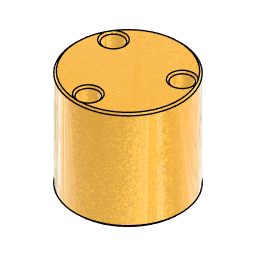
Parametric Starkiller v5 (Autodesk Fusion 360 design; units mm, degrees)
Autodesk Fusion 360 part; units mm, degrees
sketch "Sketch1" plane through (0, 0, 0) normal (0, 0, 1) x (1, 0, 0)
  circle A0 centre (0, 0) radius 11.7
  dimension "d18" = 23.4
  constraint coincident A0.centre origin
  measures "d18" diameter of A0
extrude "Main body contour" add sketch "Sketch1" along normal blind 22
sketch "bottom circle" plane through (0, 0, 0) normal (0, 0, -1) x (1, 0, 0)
  circle A0 centre (0, 0) radius 11.7
  circle A1 centre (0, 0) radius 5.69
  dimension "d21" = 11.38
  constraint concentric A0 A1
  measures "d21" diameter of A1
ref_plane "WorkPlane1" through (0, 0, 22) normal (0, 0, 1) x (1, 0, 0)
extrude "bottom hole" cut sketch "bottom circle" against normal blind 6.4 contours A1
sketch "Sketch3" plane through (0, 0, 22) normal (0, 0, 1) x (1, 0, 0)
  circle A0 centre (0, 0) radius 11.7 construction
  line L0 (0, 0) -> (0, -8.85) construction
  circle A1 centre (0, -8.85) radius 2.1
  circle A2 centre (0, 0) radius 12.6 construction
  circle A3 centre (0, 0) radius 5.1 construction
  circle A4 centre (0, -8.85) radius 3.75 construction
  dimension "d25" = 4.2
  dimension "d50" = 25.2
  dimension "d51" = 10.2
  constraint coincident A0.centre L0.start
  constraint vertical L0
  constraint coincident L0.end A1.centre
  constraint concentric A0 A3
  constraint concentric A1 A4
  constraint tangent A2 A4
  constraint tangent A3 A4
  measures "d25" diameter of A1
  measures "d50" diameter of A2
  measures "d51" diameter of A3
extrude "Extrude3" cut sketch "Sketch3" against normal blind 6.4
pattern_circular "C-Pattern1" count 3 over 360 about axis through (0, 0, 1.75) along (0, 0, 1) of "Extrude3"
sketch "Sketch4" plane through (0, 0, 0) normal (0, 0, -1) x (1, 0, 0)
  circle A0 centre (0, 0) radius 5.69
  circle A1 centre (0, 0) radius 11.7
  line L0 (0, 0) -> (0, 5.69) construction
  line L1 (-0.4202, 5.6745) -> (0, 5.29)
  line L2 (0, 5.29) -> (0.4202, 5.6745)
  line L3 (-0.4202, 5.6745) -> (0, 0) construction
  line L4 (0, 0) -> (0.4202, 5.6745) construction
  dimension "d34" = 0.4
  dimension "d43" = 8.471
  constraint coincident A0.centre A1.centre
  constraint coincident A0 L0.end
  constraint vertical L0
  constraint coincident A0 L1.start
  constraint coincident L0 L1.end
  constraint coincident A0 L2.end
  constraint equal L1 L2
  measures "d34" distance of L0.end L1.end
  measures "d43" angle of L3 L4
extrude "Extrude4" add sketch "Sketch4" against normal blind 6.4 contours A0 L1 L2 picked at (0, 5.5555)
sketch "Sketch5" plane through (0, 0, 0) normal (1, 0, 0) x (0, 1, 0)
  line L0 (-5.6745, 6.4) -> (-5.6745, 0)
  line L1 (5.69, 0) -> (-5.6745, 0)
  line L2 (-5.6745, 0) -> (-5.6745, 6.4)
  line L3 (5.69, 0) -> (5.69, 0.4) construction
  line L4 (5.69, 0.4) -> (6.09, 0)
  line L5 (5.69, 0) -> (6.09, 0)
  line L6 (5.69, 0.4) -> (5.29, 0.8)
  line L7 (5.29, 0.8) -> (5.29, 0)
  line L8 (5.69, 6.4) -> (-5.6745, 6.4)
  dimension "d46" = 0.4
  dimension "d47" = 0.4
  constraint coincident L1.start L3.start
  constraint perpendicular L1 L3
  constraint equal L3 L5
  constraint horizontal L5
  constraint parallel L4 L6
  constraint coincident L1 L7.end
  constraint perpendicular L1 L7
  measures "d46" distance of L1.start L3.end
  measures "d47" distance of L1.start L7.end
pattern_circular "C-Pattern2" count 17 over 360 about axis through (0, 0, 1.75) along (0, 0, 1) of "Extrude4"
chamfer "Chamfer1" distance 0.4 angle 45 5 edges at (-10.9082, -4.2309, 0) (-10.9082, -4.2309, 22) (-1.9579, -8.0906, 22) (-6.0277, 5.7409, 22) (7.9856, 2.3497, 22)
revolve "Revolve1" cut sketch "Sketch5" angle 360 about axis through (0, 0, 1.75) along (0, 0, 1)
equation "stages = 3"
equation "stageHeight = 6 mm"
equation "bottomStageTeeth = 17"
equation "modulus = 0.6 mm"
equation "prongDia = 4 mm"
equation "outerDia = 23.4 mm"
equation "bottomStageOuterDia = bottomStageTeeth * modulus + 2 * modulus"
equation "bottomStageHoleRadiusOffset = -0.01 mm"
equation "bottomStageHoleDia = bottomStageOuterDia + bottomStageHoleRadiusOffset * 2"
equation "stageSeparatorCount = max(0; stages - 1)"
equation "stageSeparatorSize = 2 mm"
equation "totalHeight = stages * stageHeight + stageSeparatorCount * stageSeparatorSize"
equation "prongHoleRadiusOffset = 0.1 mm"
equation "prongHoleDia = prongDia + prongHoleRadiusOffset * 2"
equation "bridgeExtraRoom = 0.4 mm"
equation "d18 = outerDia"
equation "d19 = totalHeight"
equation "d21 = bottomStageHoleDia"
equation "d22 = -stageHeight - bridgeExtraRoom"
equation "d25 = prongHoleDia"
equation "d28 = -stageHeight - bridgeExtraRoom"
equation "gearInsertHeight = 0.4 mm"
equation "d34 = gearInsertHeight"
equation "gearInsertPcOfAngle = 0.8"
equation "gearInsertWidthAngle = ( 360 * ( gearInsertPcOfAngle / 2 ) / bottomStageTeeth ) * 1 deg"
equation "d41 = bottomStageTeeth"
equation "d43 = gearInsertWidthAngle"
equation "d47 = gearInsertHeight"
equation "d49 = -min(totalHeight; stageHeight + bridgeExtraRoom)"
equation "d50 = 42 * modulus"
equation "d51 = modulus * topStageTeeth"
equation "topStageTeeth = 17"
named bodies: "Starkiller"
